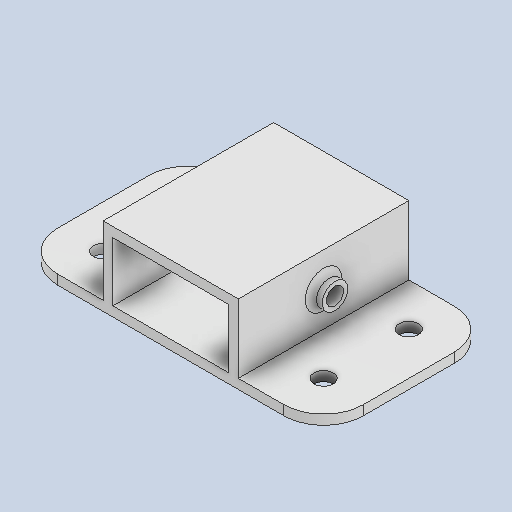
# Autodesk Inventor part: BeamHoldertoBack
Saved by Autodesk Inventor 2023 (Build 270158000, 158)
## iProperties
Created: 2022-10-18
Part Number: BeamHoldertoBack
Material: ABS Plastic
Document SubType Name: Modeling
Designer: Miner
Density: 1.06 g/cm^3
Appearance: Smooth - White
Author: Miner
Autodesk Inventor part; units mm, degrees
ref_plane "YZ Plane" through (0, 0, 0) normal (1, 0, 0) x (0, 1, 0)
ref_plane "XZ Plane" through (0, 0, 0) normal (0, 1, 0) x (-1, 0, 0)
ref_plane "XY Plane" through (0, 0, 0) normal (0, 0, 1) x (1, 0, 0)
sketch "Sketch1" plane through (0, 0, 0) normal (0, 0, 1) x (1, 0, 0)
  line L0 (-10.2, -5.2) -> (10.2, -5.2)
  line L1 (10.2, -5.2) -> (10.2, 5.2)
  line L2 (10.2, 5.2) -> (-10.2, 5.2)
  line L3 (-10.2, 5.2) -> (-10.2, -5.2)
  line L4 (-10.2, -5.2) -> (10.2, 5.2) construction
  line L5 (10.2, -5.2) -> (-10.2, 5.2) construction
  line L6 (-11.9, 6.9) -> (11.9, 6.9)
  line L7 (11.9, 6.9) -> (11.9, -6.9)
  line L8 (11.9, -6.9) -> (-11.9, -6.9)
  line L9 (-11.9, -6.9) -> (-11.9, 6.9)
  point P0 (0, 0)
  dimension "d0" = 20.4
  dimension "d1" = 10.4
  dimension "d2" = 1.7
  constraints: 20 end point, 4 parallel, 2 midpoint, 2 perpendicular, 1 horizontal, 3 other
  measures "d0" distance of L2.end L1.end
  measures "d1" distance of L1.end L0.end
  measures "d2" distance between parallel lines of L2 L6
extrude "Extrusion1" add sketch "Sketch1" along normal blind 30
sketch "Sketch2" plane through (-11.9, -6.9, 0) normal (0, -1, 0) x (1, 0, 0)
  line L0 (-15, 0) -> (38.8, 0)
  line L1 (38.8, 0) -> (38.8, 30)
  line L2 (38.8, 30) -> (-15, 30)
  line L3 (-15, 30) -> (-15, 0)
  line L4 (-15, 0) -> (38.8, 30) construction
  line L5 (38.8, 0) -> (-15, 30) construction
  point P0 (11.9, 0)
  point P1 (11.9, 15)
  dimension "d5" = 53.8
  dimension "d23" = 30
  constraints: 12 end point, 2 midpoint, 2 parallel, 1 horizontal, 1 perpendicular
  measures "d5" distance of L2.end L1.end
  measures "d23" distance of L2.end L0.start
extrude "Extrusion2" add sketch "Sketch2" against normal blind 1.7
sketch "Sketch3" plane through (-11.9, -5.2, 0) normal (0, 1, 0) x (1, 0, 0)
  line L0 (-15, 0) -> (38.8, 0) construction
  line L1 (0, 0) -> (0, -30) construction
  line L2 (-15, 0) -> (0, 0) construction
  line L3 (0, 0) -> (0, -15) construction
  line L4 (0, -15) -> (-15, -15) construction
  line L5 (-15, -15) -> (-15, 0) construction
  line L6 (-15, 0) -> (0, -15) construction
  line L7 (-15, 0) -> (-15, -30) construction
  line L8 (0, -15) -> (-15, -30) construction
  point P0 (11.9, 0)
  point P1 (-7.5, -7.5)
  point P2 (-7.5, -22.5)
  point P3 (-15, -7.5)
  point P4 (-7.5, 0)
  dimension "d24" = 7.5
  dimension "d25" = 7.5
  constraints: 12 end point, 5 midpoint, 2 parallel, 2 perpendicular, 1 horizontal
  measures "d24" distance of point (-15, -7.5) point (-7.5, -7.5)
  measures "d25" distance of point (-7.5, 0) point (-7.5, -7.5)
hole "Hole1" at (-19.4, -5.2, 7.5) at (-19.4, -5.2, 22.5) direction (0, -1, 0) diameter 3.4 depth 5 tip angle 118
mirror "Mirror1" about plane through (0, 0, 0) normal (1, 0, 0) of "Hole1"
fillet "Fillet1" radius 7 4 edges at (26.9, -6.05, 30) (26.9, -6.05, 0) (-26.9, -6.05, 0) (-26.9, -6.05, 30)
sketch "Sketch4" plane through (11.9, 6.9, 30) normal (1, 0, 0) x (0, 0, -1)
  line L0 (30, 0) -> (0, 0) construction
  line L1 (30, -12.1) -> (0, -12.1) construction
  line L2 (0, 0) -> (30, -12.1) construction
  circle A0 centre (15, -6.05) radius 1.5
  circle A1 centre (15, -6.05) radius 2.25
  point P0 (30, -6.9)
  dimension "d16" = 3
  dimension "d17" = 0.75
  constraints: 2 centre point, 2 end point, 1 coincident, 1 midpoint
  measures "d16" diameter of A0
  measures "d17" radial gap between concentric circles of A0 A1
extrude "Extrusion3" add sketch "Sketch4" along normal blind 2
fillet "Fillet2" radius 1 1 edges at (11.9, 0.85, 17.25)
extrude "Extrusion4" cut sketch "Sketch4" against normal blind 2 contours A0
body "Solid1"
